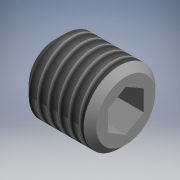
# Autodesk Inventor part: SET-SCREW12-12
Saved by Autodesk Inventor 2017.3 (Build 213256000, 256)
## iProperties
Part Number: SET-SCREW12-12
Material: Generic
Catalog Web Link: www.cadenas.de
Description: SET-SCREW-Set Screw - Flat End
Vendor: MISUMI
Document SubType Name: Modeling
Designer: partserver
Manufacturer: MISUMI
Mass: 1.11865 g
Surface Area: 7.14886 cm^2
Volume: 1.11865 cm^3
Density: 1 g/cm^3
Appearance: PSOLRGB-175-175-175
Category: PARTsolutions
Company: MISUMI
Title: SET-SCREW12-12
Author: Cadenas PARTsolutions
Comments: Set Screw - Flat End
PSOL_IDENT_0: {$CADENAS_DATA\23d-libs\misumi\metric\accessories\set_screw.prj},174 {VTYP=3D},{NB=SET-SCREW12-12},{
PSOL_IDENT_1: LINA=SET-SCREW12-12},{NN=SET-SCREW},{DATE=30.10.2020 15:47:10},{GEOMDATE=11.12.2013 00:00:00},{VERSI
PSOL_IDENT_2: ON=},{LINEID=100},{WBVAR=L},{WBNUMERIC=L}  {NB=SET-SCREW12-12},{LINA=SET-SCREW12-12},{KT=DUMMY},{PN=
PSOL_IDENT_3: SET-SCREW12-12},{TYPE=SET-SCREW},{M=12.0},{P=1.75},{L=12},{LMIN=6.6},{LALG=[6.6:42/0.1]},{B=6.0},{C=
PSOL_IDENT_4: 4.8},{DD=8.5}
NB: SET-SCREW12-12
NN: SET-SCREW
NT: Set Screw - Flat End
NBSYN: $PN.
LINA: SET-SCREW12-12
CATALOG: Misumi
PN: SET-SCREW12-12
M: 12
P: 1.75
L: 12
B: 6
C: 4.8
DD: 8.5
SUPPLIER: MISUMI
ARTICLENO: SET-SCREW12-12
BOMINFO: SET-SCREW12-12
CREATOR: CADENAS GmbH
Autodesk Inventor part; units mm, degrees
sketch "Sketch_1" plane through (0, 0, 0) normal (0, 0, 1) x (1, 0, 0)
  line L0 (0, 0) -> (-12, 0)
  line L1 (-12, 0) -> (-12, 4.9265)
  line L2 (-12, 4.9265) -> (-10.9265, 6)
  line L3 (-10.9265, 6) -> (-1.75, 6)
  line L4 (-1.75, 6) -> (0, 4.25)
  line L5 (0, 4.25) -> (0, 0)
  line L6 (0, 0) -> (-12, 0)
  constraints: 14 end point
revolve "Revolution1" add sketch "Sketch_1" angle 360 about axis through (0, 0, 0) along (1, 0, 0)
thread "Thread1" size "M12x1.75" class "6g" standard "ISO Metric profile" full length
sketch "Sketch_2" plane through (-12, 0, 0) normal (-1, 0, 0) x (0, 1, 0)
  line L0 (-3, -1.7321) -> (0, -3.4641)
  line L1 (0, -3.4641) -> (3, -1.7321)
  line L2 (3, -1.7321) -> (3, 1.7321)
  line L3 (3, 1.7321) -> (0, 3.4641)
  line L4 (0, 3.4641) -> (-3, 1.7321)
  line L5 (-3, 1.7321) -> (-3, -1.7321)
  constraints: 12 end point
extrude "Extrusion1" cut sketch "Sketch_2" against normal blind 4.8
sketch "Sketch_3" plane through (0, 0, 0) normal (0, 0, 1) x (1, 0, 0)
  line L0 (-5.4679, 0) -> (-7.2, 0)
  line L1 (-7.2, 0) -> (-7.2, 3)
  line L2 (-7.2, 3) -> (-5.4679, 0)
  line L3 (-5.4679, 0) -> (-7.2, 0)
  constraints: 8 end point
revolve "Revolution2" cut sketch "Sketch_3" angle 360 about axis through (-5.4679, 0, 0) along (1, 0, 0)
ref_plane "CP_XY" through (0, 0, 0) normal (1, 0, 0) x (0, 0, -1)
ref_plane "CP_YZ" through (0, 0, 0) normal (0, 0, -1) x (0, 1, 0)
ref_plane "CP_ZX" through (0, 0, 0) normal (0, 1, 0) x (1, 0, 0)
body "Solid1"
